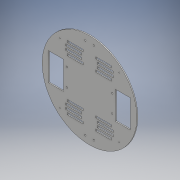
# Autodesk Inventor part: Base
Saved by Autodesk Inventor 2018 (Build 220112000, 112)
## iProperties
Created: 2018-02-22
Part Number: Base
Material: Genérico
Document SubType Name: Modeling
Designer: ivanb
Density: 1 g/cm^3
Appearance: Valor por defecto
Author: ivanb
Autodesk Inventor part; units mm, degrees
ref_plane "YZ Plane" through (0, 0, 0) normal (1, 0, 0) x (0, 1, 0)
ref_plane "XZ Plane" through (0, 0, 0) normal (0, 1, 0) x (-1, 0, 0)
ref_plane "XY Plane" through (0, 0, 0) normal (0, 0, 1) x (1, 0, 0)
sketch "Boceto1" plane through (0, 0, 0) normal (0, 1, 0) x (-1, 0, 0)
  circle A0 centre (0, 0) radius 75
  line L0 (65, -22) -> (41, -22)
  line L1 (41, -22) -> (41, 22)
  line L2 (41, 22) -> (65, 22)
  line L3 (65, 22) -> (65, -22)
  line L4 (37.6072, -39) -> (12.6072, -39)
  line L5 (12.6072, -39) -> (12.6072, -36)
  line L6 (12.6072, -36) -> (37.6072, -36)
  line L7 (37.6072, -36) -> (37.6072, -39)
  line L8 (37.6072, -45) -> (12.6072, -45)
  line L9 (12.6072, -45) -> (12.6072, -42)
  line L10 (12.6072, -42) -> (37.6072, -42)
  line L11 (37.6072, -42) -> (37.6072, -45)
  line L12 (35, -51) -> (10, -51)
  line L13 (10, -51) -> (10, -48)
  line L14 (10, -48) -> (35, -48)
  line L15 (35, -48) -> (35, -51)
  line L16 (35, -33) -> (10, -33)
  line L17 (10, -33) -> (10, -30)
  line L18 (10, -30) -> (35, -30)
  line L19 (35, -30) -> (35, -33)
  line L20 (-37.6072, -39) -> (-12.6072, -39)
  line L21 (-12.6072, -39) -> (-12.6072, -36)
  line L22 (-12.6072, -36) -> (-37.6072, -36)
  line L23 (-37.6072, -36) -> (-37.6072, -39)
  line L24 (-37.6072, -45) -> (-12.6072, -45)
  line L25 (-37.6072, -42) -> (-37.6072, -45)
  line L26 (-12.6072, -42) -> (-37.6072, -42)
  line L27 (-12.6072, -45) -> (-12.6072, -42)
  line L28 (-35, -51) -> (-10, -51)
  line L29 (-35, -48) -> (-35, -51)
  line L30 (-10, -48) -> (-35, -48)
  line L31 (-10, -51) -> (-10, -48)
  line L32 (-35, -33) -> (-10, -33)
  line L33 (-35, -30) -> (-35, -33)
  line L34 (-10, -30) -> (-35, -30)
  line L35 (-10, -33) -> (-10, -30)
  line L36 (-65, -22) -> (-41, -22)
  line L37 (-41, -22) -> (-41, 22)
  line L38 (-41, 22) -> (-65, 22)
  line L39 (-65, 22) -> (-65, -22)
  line L40 (37.6072, 39) -> (12.6072, 39)
  line L41 (12.6072, 39) -> (12.6072, 36)
  line L42 (12.6072, 36) -> (37.6072, 36)
  line L43 (37.6072, 36) -> (37.6072, 39)
  line L44 (37.6072, 45) -> (12.6072, 45)
  line L45 (37.6072, 42) -> (37.6072, 45)
  line L46 (12.6072, 42) -> (37.6072, 42)
  line L47 (12.6072, 45) -> (12.6072, 42)
  line L48 (35, 51) -> (10, 51)
  line L49 (35, 48) -> (35, 51)
  line L50 (10, 48) -> (35, 48)
  line L51 (10, 51) -> (10, 48)
  line L52 (35, 33) -> (10, 33)
  line L53 (35, 30) -> (35, 33)
  line L54 (10, 30) -> (35, 30)
  line L55 (10, 33) -> (10, 30)
  line L56 (-35, 30) -> (-35, 33)
  line L57 (-10, 33) -> (-10, 30)
  line L58 (-10, 30) -> (-35, 30)
  line L59 (-35, 33) -> (-10, 33)
  line L60 (-12.6072, 39) -> (-12.6072, 36)
  line L61 (-12.6072, 36) -> (-37.6072, 36)
  line L62 (-37.6072, 36) -> (-37.6072, 39)
  line L63 (-37.6072, 39) -> (-12.6072, 39)
  line L64 (-12.6072, 45) -> (-12.6072, 42)
  line L65 (-12.6072, 42) -> (-37.6072, 42)
  line L66 (-37.6072, 45) -> (-12.6072, 45)
  line L67 (-10, 48) -> (-35, 48)
  line L68 (-35, 51) -> (-10, 51)
  line L69 (-10, 51) -> (-10, 48)
  line L70 (-37.6072, 42) -> (-37.6072, 45)
  line L71 (-35, 48) -> (-35, 51)
  point P0 (0, 25.3749)
  dimension "d0" = 150
  dimension "d1" = 24
  dimension "d2" = 44
  dimension "d3" = 10
  dimension "d4" = 25
  dimension "d5" = 3
  dimension "d6" = 25
  dimension "d7" = 3
  dimension "d8" = 25
  dimension "d9" = 3
  dimension "d10" = 25
  dimension "d11" = 3
  dimension "d12" = 3
  dimension "d13" = 3
  dimension "d14" = 3
  dimension "d15" = 0
  constraints: 144 end point, 10 parallel, 5 horizontal, 5 perpendicular, 1 centre point
  measures "d0" diameter of A0
  measures "d1" distance of L1.end L2.end
  measures "d2" distance of L0.end L1.end
  measures "d3" distance edge to line of A0 L3
  measures "d4" distance of L5.end L6.end
  measures "d5" distance of L4.end L5.end
  measures "d6" distance of L10.start L11.start
  measures "d7" distance of L8.end L10.start
  measures "d8" distance of L14.start L15.start
  measures "d9" distance of L12.end L14.start
  measures "d10" distance of L18.start L19.start
  measures "d11" distance of L16.end L18.start
  measures "d12" distance between parallel lines of L8 L14
  measures "d13" distance between parallel lines of L4 L10
  measures "d14" distance between parallel lines of L16 L6
  measures "d15" distance between parallel lines of L13 L17
extrude "Extrusión1" add sketch "Boceto1" along normal blind 1.5
sketch "Boceto2" plane through (0, 1.5, 0) normal (0, 1, 0) x (1, 0, 0)
  line L0 (0, 0) -> (0, -9.9603)
  line L1 (0, 0) -> (61.7788, -62.8893)
  circle A0 centre (47.0174, -47.8626) radius 0.75
  arc A1 (50.5529, -44.327) -> (43.5135, -51.4295) centre (47.0174, -47.8626) ccw
  line L2 (-72.438, 0) -> (-75, 0)
  circle A2 centre (0, 0) radius 72.438
  line L3 (44.0781, -44.8705) -> (47.0174, -47.8626)
  line L4 (43.4505, -51.3665) -> (48.0344, -55.9504)
  line L5 (43.4505, -51.3665) -> (49.9332, -51.3665) construction
  line L6 (47.0174, -47.8626) -> (52.0174, -47.8626) construction
  line L7 (50.5529, -44.327) -> (55.1054, -48.8795)
  line L8 (55.1054, -48.8795) -> (48.0344, -55.9504)
  circle A3 centre (-47.0174, -47.8626) radius 0.75
  arc A4 (-43.5135, -51.4295) -> (-50.5529, -44.327) centre (-47.0174, -47.8626) ccw
  line L9 (-44.0781, -44.8705) -> (-47.0174, -47.8626)
  line L10 (-43.4505, -51.3665) -> (-48.0344, -55.9504)
  line L11 (-43.4505, -51.3665) -> (-49.9332, -51.3665) construction
  line L12 (-47.0174, -47.8626) -> (-52.0174, -47.8626) construction
  line L13 (-50.5529, -44.327) -> (-55.1054, -48.8795)
  line L14 (-55.1054, -48.8795) -> (-48.0344, -55.9504)
  line L15 (0, 0) -> (7.916, 0)
  line L16 (-44.0781, 44.8705) -> (-47.0174, 47.8626)
  circle A5 centre (-47.0174, 47.8626) radius 0.75
  line L17 (-43.4505, 51.3665) -> (-49.9332, 51.3665) construction
  arc A6 (-50.5529, 44.327) -> (-43.5135, 51.4295) centre (-47.0174, 47.8626) ccw
  line L18 (-43.4505, 51.3665) -> (-48.0344, 55.9504)
  line L19 (-47.0174, 47.8626) -> (-52.0174, 47.8626) construction
  line L20 (-50.5529, 44.327) -> (-55.1054, 48.8795)
  line L21 (-55.1054, 48.8795) -> (-48.0344, 55.9504)
  line L22 (0, 0) -> (61.7788, 62.8893)
  circle A7 centre (0, 0) radius 72.438
  circle A8 centre (47.0174, 47.8626) radius 0.75
  arc A9 (43.5135, 51.4295) -> (50.5529, 44.327) centre (47.0174, 47.8626) ccw
  line L23 (44.0781, 44.8705) -> (47.0174, 47.8626)
  line L24 (43.4505, 51.3665) -> (48.0344, 55.9504)
  line L25 (47.0174, 47.8626) -> (52.0174, 47.8626) construction
  line L26 (55.1054, 48.8795) -> (48.0344, 55.9504)
  line L27 (50.5529, 44.327) -> (55.1054, 48.8795)
  line L28 (43.4505, 51.3665) -> (49.9332, 51.3665) construction
  dimension "d26" = 1.5
  dimension "d27" = 45
  dimension "d28" = 44.49
  dimension "d29" = 45.51
  constraints: 58 end point, 31 symmetric about line, 12 point on circle, 9 centre point, 8 point on line, 6 coincident, 3 horizontal, 1 collinear, 1 equal length, 1 horizontal alignment, 1 line through centre, 1 perpendicular, 1 tangent, 8 other
  measures "d26" diameter of A0
  measures "d27" angle of L4 L5
  measures "d28" angle of L1 L0
  measures "d29" angle of L1 L15
extrude "Extrusión2" cut sketch "Boceto2" against normal blind 10 contours A0 L1 | L1 A0 | A8 L22 | L22 A8 | A3 | A5
sketch "Boceto3" plane through (0, 0, 0) normal (0, -1, 0) x (1, 0, 0)
  line L0 (0, 0) -> (0, 96.9999)
  line L1 (0, 0) -> (57.8177, 0)
  circle A0 centre (6.75, 65) radius 1.25
  circle A1 centre (-6.75, 65) radius 1.25
  circle A2 centre (6.75, -65) radius 1.25
  circle A3 centre (-6.75, -65) radius 1.25
  dimension "d32" = 2.5
  dimension "d33" = 6.75
  dimension "d34" = 65
  constraints: 4 centre point, 4 end point, 3 symmetric about line, 1 horizontal, 1 vertical, 3 other
  measures "d32" diameter of A0
  measures "d33" distance from line of L0 A0.centre
  measures "d34" distance from line of L1 A0.centre
extrude "Extrusión3" cut sketch "Boceto3" against normal blind 10
sketch "Boceto4" plane through (0, 0, 0) normal (0, -1, 0) x (1, 0, 0)
  circle A0 centre (-36, 14) radius 1.25
  line L0 (0, 0) -> (0, 13.2611)
  line L1 (0, 0) -> (12.4525, 0)
  circle A1 centre (36, 14) radius 1.25
  circle A2 centre (-36, -14) radius 1.25
  circle A3 centre (36, -14) radius 1.25
  line L2 (-41, 22) -> (-41, -22) projected
  point P0 (0, -13.2611)
  dimension "d37" = 2.5
  dimension "d38" = 14
  dimension "d39" = 5
  constraints: 4 centre point, 4 end point, 4 symmetric about line, 1 horizontal, 1 vertical, 3 other
  measures "d37" diameter of A0
  measures "d38" distance from line of L1 A0.centre
  measures "d39" distance from line of L2 A0.centre
extrude "Extrusión4" cut sketch "Boceto4" against normal blind 10
